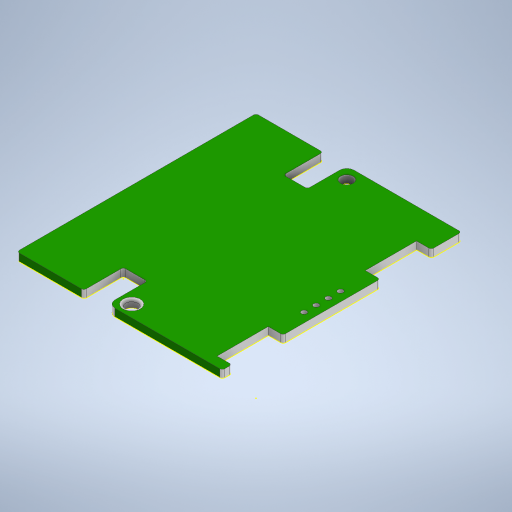
# Autodesk Inventor part: PCB_GORNE
Saved by Autodesk Inventor 2023 (Build 270158000, 158)
## iProperties
Created: 2023-12-23
Part Number: PCB_GORNE
Material: Ogólny
Document SubType Name: Modeling
Designer: Kamil
Density: 1 g/cm^3
Appearance: Domyślna
Author: Kamil
Autodesk Inventor part; units mm, degrees
ref_plane "YZ Plane" through (0, 0, 0) normal (1, 0, 0) x (0, 1, 0)
ref_plane "XZ Plane" through (0, 0, 0) normal (0, 1, 0) x (-1, 0, 0)
ref_plane "XY Plane" through (0, 0, 0) normal (0, 0, 1) x (1, 0, 0)
sketch "Szkic1" plane through (0, 0, 0) normal (0, 1, 0) x (-1, 0, 0)
  line L0 (0, 0) -> (50, 0)
  line L1 (50, 0) -> (50, -50)
  line L2 (50, -50) -> (0, -50)
  line L3 (0, -50) -> (0, 0)
  dimension "d0" = 50
  dimension "d1" = 50
  constraints: 8 end point, 2 parallel, 1 horizontal, 1 perpendicular
  measures "d0" distance of L1.end L2.end
  measures "d1" distance of L0.end L1.end
extrude "Wyciągnięcie proste1" add sketch "Szkic1" along normal blind 1.6
sketch "Szkic2" plane through (-50, 0, 0) normal (0, 0, 1) x (1, 0, 0)
  line L0 (0, 0) -> (50, 0) projected
  line L1 (50, 0) -> (50, 1.6) projected
  line L2 (0, 1.6) -> (50, 1.6) projected
  line L3 (0, 0) -> (0, 1.6) projected
  line L4 (47.9294, 17.85) -> (42.5705, -2.15) projected
  line L5 (42.5705, -2.15) -> (44.641, -2.15) projected
  line L6 (44.641, -2.15) -> (50, 17.85) projected
  line L7 (50, 17.85) -> (47.9294, 17.85) projected
  point P0 (43.5753, 1.6)
  point P1 (43.1466, 0)
extrude "Wyciągnięcie proste2" cut sketch "Szkic2" against normal through all contours L4 L2 L6 L0 | L6 L2 L1 L0
sketch "Szkic3" plane through (0, 0, 0) normal (0, -1, 0) x (1, 0, 0)
  line L0 (-8.5941, -2) -> (-8.5941, -12.7) projected
  line L1 (-8.5941, -2) -> (-10.1396, -2) projected
  line L2 (-10.1396, -12.7) -> (-10.1396, -2) projected
  line L3 (-8.5941, -12.7) -> (-10.1396, -12.7) projected
  line L4 (-10.1396, -12.7) -> (-7.8396, -12.7)
  line L5 (-7.8396, -12.7) -> (-7.8396, -2)
  line L6 (-7.8396, -2) -> (-10.1396, -2)
  line L7 (-10.1396, -2) -> (-10.1396, -12.7)
  line L8 (-8.5941, -33) -> (-8.5941, -43.7) projected
  line L9 (-8.5941, -33) -> (-10.1396, -33) projected
  line L10 (-10.1396, -43.7) -> (-10.1396, -33) projected
  line L11 (-8.5941, -43.7) -> (-10.1396, -43.7) projected
  line L12 (-10.1396, -33) -> (-7.8396, -33)
  line L13 (-7.8396, -33) -> (-7.8396, -43.7)
  line L14 (-7.8396, -43.7) -> (-10.1396, -43.7)
  line L15 (-10.1396, -43.7) -> (-10.1396, -33)
  point P0 (0, 0)
  dimension "d6" = 2.3
  dimension "d7" = 2.3
  constraints: 16 end point, 4 parallel, 2 horizontal, 2 perpendicular
  measures "d6" distance of L6.end L5.end
  measures "d7" distance of L13.end L14.end
extrude "Wyciągnięcie proste3" cut sketch "Szkic3" against normal through all
sketch "Szkic4" plane through (0, 0, 0) normal (0, -1, 0) x (1, 0, 0)
  line L0 (-10.1396, -33) -> (-7.8396, -33) projected
  line L1 (-7.8396, -12.7) -> (-10.1396, -12.7) projected
  line L2 (-8.9896, -12.7) -> (-8.9896, -33) construction
  circle A0 centre (-8.9896, -26.66) radius 0.55
  circle A1 centre (-8.9896, -24.12) radius 0.55
  circle A2 centre (-8.9896, -21.58) radius 0.55
  circle A3 centre (-8.9896, -19.04) radius 0.55
  point P0 (0, 0)
  dimension "d10" = 1.1
  dimension "d14" = 2.54
  dimension "d19" = 6.34
  constraints: 4 centre point, 2 end point, 2 midpoint, 1 point on line, 1 vertical, 6 other
  measures "d10" diameter of A0
  measures "d14" distance of A0.centre A1.centre
  measures "d19" distance from line of L0 A0.centre
extrude "Wyciągnięcie proste4" cut sketch "Szkic4" against normal through all
sketch "Szkic5" plane through (0, 0, 0) normal (0, -1, 0) x (1, 0, 0)
  line L0 (-50, -50) -> (-50, 0) projected
  circle A0 centre (-8.9896, -21.58) radius 0.55 projected
  circle A1 centre (-8.9896, -24.12) radius 0.55 projected
  circle A2 centre (-8.9896, -19.04) radius 0.55 projected
  circle A3 centre (-8.9896, -26.66) radius 0.55 projected
  line L1 (-10.1396, -12.7) -> (-10.1396, -2) projected
  line L2 (-10.1396, -2) -> (-7.8396, -2) projected
  line L3 (-7.8396, -2) -> (-7.8396, -12.7) projected
  line L4 (-7.8396, -12.7) -> (-10.1396, -12.7) projected
  line L5 (-10.1396, -43.7) -> (-10.1396, -33) projected
  line L6 (-10.1396, -33) -> (-7.8396, -33) projected
  line L7 (-7.8396, -33) -> (-7.8396, -43.7) projected
  line L8 (-7.8396, -43.7) -> (-10.1396, -43.7) projected
  line L9 (-6.8534, -50) -> (-6.8534, 0) projected
  line L10 (-50, 0) -> (-6.8534, 0) projected
  line L11 (-50, -50) -> (-50, 0) projected
  line L12 (-6.8534, -50) -> (-50, -50) projected
  line L13 (-50, -50) -> (-50, 0) projected
  line L14 (-50, -25) -> (-6.8534, -25)
  line L15 (-34, -48.25) -> (-34, -43.25) projected
  line L16 (-32, -48.25) -> (-34, -48.25) projected
  line L17 (-32, -43.25) -> (-32, -48.25) projected
  line L18 (-34, -43.25) -> (-32, -43.25) projected
  line L19 (-30.5, -46.7732) -> (-30.5, -50) projected
  line L20 (-36, -50) -> (-50, -50) projected
  line L21 (-28, -36) -> (-45.016, -36) projected
  line L22 (-30.5, -50) -> (-36, -50)
  line L23 (-36, -50) -> (-36, -41.75)
  line L24 (-36, -41.75) -> (-30.5, -41.75)
  line L25 (-30.5, -41.75) -> (-30.5, -50)
  line L26 (-36, 0) -> (-36, -8.25)
  line L27 (-36, -8.25) -> (-30.5, -8.25)
  line L28 (-30.5, -8.25) -> (-30.5, 0)
  point P0 (0, 0)
  dimension "d22" = 2
  dimension "d23" = 1.5
  constraints: 16 end point, 4 symmetric about line, 2 midpoint, 2 parallel, 1 horizontal, 1 perpendicular
  measures "d22" distance between parallel lines of L15 L23
  measures "d23" distance between parallel lines of L18 L24
extrude "Wyciągnięcie proste5" cut sketch "Szkic5" against normal through all contours L23 L24 L25 L19 L12 | L10 L28 L27 L26 | L15 L18 L17 L16
fillet "Zaokrąglenie2" radius 0.5 2 edges at (-50, 0.8, 0) (-50, 0.8, -50)
sketch "Szkic7" plane through (-6.8534, 0, -50) normal (0, 0, -1) x (-1, 0, 0)
  line L0 (-0.4287, 1.6) -> (23.6466, 1.6) projected
  line L1 (-0.4287, 1.6) -> (0, 0) projected
  line L2 (0, 0) -> (23.6466, 0) projected
  line L3 (0, 0) -> (0, 1.6)
  line L4 (0.2, 1.6) -> (0.2, 0)
  line L5 (23.6466, 0) -> (23.6466, 1.6) projected
  line L6 (42.6466, 1.6) -> (42.6466, 0) projected
  line L7 (29.1466, 1.6) -> (42.6466, 1.6) projected
  line L8 (29.1466, 1.6) -> (29.1466, 0) projected
  line L9 (29.1466, 0) -> (42.6466, 0) projected
  point P0 (-6.8534, 0)
  dimension "d30" = 0.2
  constraints: 4 end point, 3 point on line, 2 perpendicular
  measures "d30" distance between parallel lines of L3 L4
extrude "Wyciągnięcie proste7" cut sketch "Szkic7" against normal through all contours L0 L3 L1 | L0 L4 L2 L3
sketch "Szkic9" plane through (0, 1.6, 0) normal (0, 1, 0) x (1, 0, 0)
  circle A0 centre (-8.9896, 21.58) radius 0.55 projected
  circle A1 centre (-8.9896, 24.12) radius 0.55 projected
  circle A2 centre (-8.9896, 19.04) radius 0.55 projected
  circle A3 centre (-8.9896, 26.66) radius 0.55 projected
  line L0 (-10.1396, 2) -> (-10.1396, 12.7) projected
  line L1 (-10.1396, 12.7) -> (-7.8396, 12.7) projected
  line L2 (-7.8396, 12.7) -> (-7.8396, 2) projected
  line L3 (-7.8396, 2) -> (-10.1396, 2) projected
  line L4 (-10.1396, 33) -> (-10.1396, 43.7) projected
  line L5 (-10.1396, 43.7) -> (-7.8396, 43.7) projected
  line L6 (-7.8396, 43.7) -> (-7.8396, 33) projected
  line L7 (-7.8396, 33) -> (-10.1396, 33) projected
  line L8 (-7.0534, 0) -> (-7.0534, 50) projected
  line L9 (-7.0534, 50) -> (-30.5, 50) projected
  line L10 (-30.5, 50) -> (-30.5, 41.75) projected
  line L11 (-30.5, 41.75) -> (-36, 41.75) projected
  line L12 (-36, 41.75) -> (-36, 50) projected
  line L13 (-36, 50) -> (-49.5, 50) projected
  arc A4 (-49.5, 50) -> (-50, 49.5) centre (-49.5, 49.5) ccw projected
  line L14 (-50, 49.5) -> (-50, 0.5) projected
  arc A5 (-50, 0.5) -> (-49.5, 0) centre (-49.5, 0.5) ccw projected
  line L15 (-49.5, 0) -> (-36, 0) projected
  line L16 (-36, 0) -> (-36, 8.25) projected
  line L17 (-36, 8.25) -> (-30.5, 8.25) projected
  line L18 (-30.5, 8.25) -> (-30.5, 0) projected
  line L19 (-30.5, 0) -> (-7.0534, 0) projected
  line L20 (-10.1396, 12.7) -> (-7.0534, 12.7)
  line L21 (-7.0534, 12.7) -> (-7.0534, 2)
  line L22 (-7.0534, 2) -> (-10.1396, 2)
  line L23 (-10.1396, 2) -> (-10.1396, 12.7)
  line L24 (-10.1396, 43.7) -> (-7.0534, 43.7)
  line L25 (-7.0534, 43.7) -> (-7.0534, 33)
  line L26 (-7.0534, 33) -> (-10.1396, 33)
  line L27 (-10.1396, 33) -> (-10.1396, 43.7)
  point P0 (0, 0)
  point P1 (-7.8396, 2)
  constraints: 16 end point, 4 parallel, 2 horizontal, 2 perpendicular, 2 point on line
extrude "Wyciągnięcie proste8" cut sketch "Szkic9" against normal through all contours L2 L20 L8 L22 | L26 L6 L24 L8
fillet "Zaokrąglenie3" radius 0.5 6 edges at (-7.0534, 0.8, -12.7) (-7.0534, 0.8, -33) (-7.0534, 0.8, -43.7) (-7.0534, 0.8, -50) (-7.0534, 0.8, -2) (-7.0534, 0.8, 0)
sketch "Szkic11" plane through (0, 0, 0) normal (0, -1, 0) x (1, 0, 0)
  arc A0 (-7.0534, -0.5) -> (-7.5534, 0) centre (-7.5534, -0.5) ccw projected
  line L0 (-30.5, 0) -> (-7.5534, 0) projected
  line L1 (-30.5, 0) -> (-30.5, -8.25) projected
  line L2 (-30.5, -8.25) -> (-36, -8.25) projected
  line L3 (-36, -8.25) -> (-36, 0) projected
  line L4 (-49.5, 0) -> (-36, 0) projected
  arc A1 (-49.5, 0) -> (-50, -0.5) centre (-49.5, -0.5) ccw projected
  line L5 (-50, -49.5) -> (-50, -0.5) projected
  arc A2 (-50, -49.5) -> (-49.5, -50) centre (-49.5, -49.5) ccw projected
  line L6 (-36, -50) -> (-49.5, -50) projected
  line L7 (-36, -50) -> (-36, -41.75) projected
  line L8 (-36, -41.75) -> (-30.5, -41.75) projected
  line L9 (-30.5, -41.75) -> (-30.5, -50) projected
  line L10 (-7.5534, -50) -> (-30.5, -50) projected
  arc A3 (-7.5534, -50) -> (-7.0534, -49.5) centre (-7.5534, -49.5) ccw projected
  line L11 (-7.0534, -49.5) -> (-7.0534, -44.2) projected
  arc A4 (-7.0534, -44.2) -> (-7.5534, -43.7) centre (-7.5534, -44.2) ccw projected
  line L12 (-7.5534, -43.7) -> (-10.1396, -43.7) projected
  line L13 (-10.1396, -43.7) -> (-10.1396, -33) projected
  line L14 (-10.1396, -33) -> (-7.5534, -33) projected
  arc A5 (-7.5534, -33) -> (-7.0534, -32.5) centre (-7.5534, -32.5) ccw projected
  line L15 (-7.0534, -32.5) -> (-7.0534, -13.2) projected
  arc A6 (-7.0534, -13.2) -> (-7.5534, -12.7) centre (-7.5534, -13.2) ccw projected
  line L16 (-7.5534, -12.7) -> (-10.1396, -12.7) projected
  line L17 (-10.1396, -12.7) -> (-10.1396, -2) projected
  line L18 (-10.1396, -2) -> (-7.5534, -2) projected
  arc A7 (-7.5534, -2) -> (-7.0534, -1.5) centre (-7.5534, -1.5) ccw projected
  line L19 (-7.0534, -1.5) -> (-7.0534, -0.5) projected
  circle A8 centre (-8.9896, -26.66) radius 0.55 projected
  circle A9 centre (-8.9896, -19.04) radius 0.55 projected
  circle A10 centre (-8.9896, -24.12) radius 0.55 projected
  circle A11 centre (-8.9896, -21.58) radius 0.55 projected
  line L20 (-30.5, 0) -> (-31, 0)
  line L21 (-31, 0) -> (-31, -8.25)
  line L22 (-31, -8.25) -> (-30.5, -8.25)
  line L23 (-30.5, -8.25) -> (-30.5, 0)
  line L24 (-30.5, -50) -> (-31, -50)
  line L25 (-31, -50) -> (-31, -41.75)
  line L26 (-31, -41.75) -> (-30.5, -41.75)
  line L27 (-30.5, -41.75) -> (-30.5, -50)
  point P0 (0, 0)
  dimension "d40" = 0.5
  dimension "d41" = 0.5
  constraints: 16 end point, 4 parallel, 2 horizontal, 2 perpendicular, 2 point on line
  measures "d40" distance of L22.end L21.end
  measures "d41" distance of L25.end L26.end
extrude "Wyciągnięcie proste10" add sketch "Szkic11" against normal up to surface (1.6 mm away) contours L1 L2 L21 L20 | L8 L9 L24 L25
fillet "Zaokrąglenie4" radius 1.5 2 edges at (-31, 0.8, -50) (-31, 0.8, 0)
fillet "Zaokrąglenie5" radius 0.5 6 edges at (-31, 0.8, -8.25) (-36, 0.8, -8.25) (-36, 0.8, 0) (-36, 0.8, -50) (-36, 0.8, -41.75) (-31, 0.8, -41.75)
sketch "Szkic13" plane through (0, 0, 0) normal (0, -1, 0) x (1, 0, 0)
  circle A0 centre (-28.5, -2.5) radius 1 projected
  circle A1 centre (-28.5, -47.5) radius 1 projected
  point P0 (0, 0)
hole "Otwór2" at (-28.5, 0, -2.5) at (-28.5, 0, -47.5) direction (0, 1, 0) diameter 2.6 end through all
fillet "Zaokrąglenie6" radius 0.5 1 edges at (-28.5, 1.6, -1.2)
sketch "Szkic14" plane through (0, 0, 0) normal (0, -1, 0) x (1, 0, 0)
  circle A0 centre (-28.5, -2.5) radius 1.3 projected
  circle A1 centre (-28.5, -47.5) radius 1.3 projected
  arc A2 (-36.5, -50) -> (-36, -49.5) centre (-36.5, -49.5) ccw projected
  line L0 (-36, -49.5) -> (-36, -42.25) projected
  arc A3 (-35.5, -41.75) -> (-36, -42.25) centre (-35.5, -42.25) ccw projected
  line L1 (-35.5, -41.75) -> (-31.5, -41.75) projected
  arc A4 (-31, -42.25) -> (-31.5, -41.75) centre (-31.5, -42.25) ccw projected
  line L2 (-31, -42.25) -> (-31, -48.5) projected
  arc A5 (-31, -48.5) -> (-29.5, -50) centre (-29.5, -48.5) ccw projected
  line L3 (-29.5, -50) -> (-7.5534, -50) projected
  arc A6 (-7.5534, -50) -> (-7.0534, -49.5) centre (-7.5534, -49.5) ccw projected
  line L4 (-7.0534, -49.5) -> (-7.0534, -44.2) projected
  arc A7 (-7.0534, -44.2) -> (-7.5534, -43.7) centre (-7.5534, -44.2) ccw projected
  line L5 (-7.5534, -43.7) -> (-10.1396, -43.7) projected
  line L6 (-10.1396, -43.7) -> (-10.1396, -33) projected
  line L7 (-10.1396, -33) -> (-7.5534, -33) projected
  arc A8 (-7.5534, -33) -> (-7.0534, -32.5) centre (-7.5534, -32.5) ccw projected
  line L8 (-7.0534, -32.5) -> (-7.0534, -13.2) projected
  arc A9 (-7.0534, -13.2) -> (-7.5534, -12.7) centre (-7.5534, -13.2) ccw projected
  line L9 (-7.5534, -12.7) -> (-10.1396, -12.7) projected
  line L10 (-10.1396, -12.7) -> (-10.1396, -2) projected
  line L11 (-10.1396, -2) -> (-7.5534, -2) projected
  arc A10 (-7.5534, -2) -> (-7.0534, -1.5) centre (-7.5534, -1.5) ccw projected
  line L12 (-7.0534, -1.5) -> (-7.0534, -0.5) projected
  arc A11 (-7.0534, -0.5) -> (-7.5534, 0) centre (-7.5534, -0.5) ccw projected
  line L13 (-29.5, 0) -> (-7.5534, 0) projected
  arc A12 (-29.5, 0) -> (-31, -1.5) centre (-29.5, -1.5) ccw projected
  line L14 (-31, -1.5) -> (-31, -7.75) projected
  arc A13 (-31.5, -8.25) -> (-31, -7.75) centre (-31.5, -7.75) ccw projected
  line L15 (-31.5, -8.25) -> (-35.5, -8.25) projected
  arc A14 (-36, -7.75) -> (-35.5, -8.25) centre (-35.5, -7.75) ccw projected
  line L16 (-36, -7.75) -> (-36, -0.5) projected
  arc A15 (-36, -0.5) -> (-36.5, 0) centre (-36.5, -0.5) ccw projected
  line L17 (-49.5, 0) -> (-36.5, 0) projected
  arc A16 (-49.5, 0) -> (-50, -0.5) centre (-49.5, -0.5) ccw projected
  line L18 (-50, -49.5) -> (-50, -0.5) projected
  arc A17 (-50, -49.5) -> (-49.5, -50) centre (-49.5, -49.5) ccw projected
  line L19 (-36.5, -50) -> (-49.5, -50) projected
  circle A18 centre (-8.9896, -21.58) radius 0.55 projected
  circle A19 centre (-8.9896, -24.12) radius 0.55 projected
  circle A20 centre (-8.9896, -19.04) radius 0.55 projected
  circle A21 centre (-8.9896, -26.66) radius 0.55 projected
  point P0 (0, 0)
